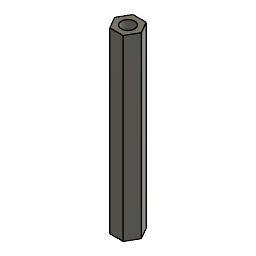
mid360_platform_standoff_v0_1 (Autodesk Fusion 360 design; units mm, degrees)
part number: 2026-06-01-18-58-21-788
Autodesk Fusion 360 part; units mm, degrees
sketch "草图1" plane through (0, 0, 0) normal (0, 1, 0) x (1, 0, 0)
  line L0 (-1.5, -2.5981) -> (1.5, -2.5981)
  line L1 (1.5, -2.5981) -> (3, 0)
  line L2 (3, 0) -> (1.5, 2.5981)
  line L3 (1.5, 2.5981) -> (-1.5, 2.5981)
  line L4 (-1.5, 2.5981) -> (-3, 0)
  line L5 (-3, 0) -> (-1.5, -2.5981)
  dimension "d2" = 5.1962
  constraint horizontal L0
  measures "d2" distance of L0 L3
sketch "草图2" plane through (0, 0, 0) normal (0, 1, 0) x (1, 0, 0)
extrude "拉伸1" add sketch "草图1" along normal blind 50
sketch "草图3" plane through (0, 50, 0) normal (0, 1, 0) x (-1, 0, 0)
  line L0 (3, 0) -> (1.5, 2.5981)
  line L1 (1.5, 2.5981) -> (-1.5, 2.5981)
  line L2 (-1.5, 2.5981) -> (-3, 0)
  line L3 (-3, 0) -> (-1.5, -2.5981)
  line L4 (-1.5, -2.5981) -> (1.5, -2.5981)
  line L5 (1.5, -2.5981) -> (3, 0)
  circle A0 centre (0, 0) radius 1.5
  dimension "d5" = 3
  constraint coincident A0.centre origin
  measures "d5" diameter of A0
extrude "拉伸2" cut sketch "草图3" against normal blind 40 contours A0
extrude "拉伸3" cut 1 faces at (-0.0374, 50, -2.2307) along direction (0, -1, 0) blind 10
